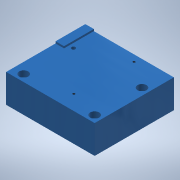
# Autodesk Inventor part: baseblock for AOTF
Saved by Autodesk Inventor 2022 (Build 260153000, 153)
## iProperties
Created: 2013-10-25
Part Number: baseblock for AOTF
Document SubType Name: Modeling
Designer: betzige
Density: 1 g/cm^3
Material: Generic
Appearance: Cyan
Author: betzige
Autodesk Inventor part; units mm, degrees
ref_plane "YZ Plane" through (0, 0, 0) normal (1, 0, 0) x (0, 1, 0)
ref_plane "XZ Plane" through (0, 0, 0) normal (0, 1, 0) x (-1, 0, 0)
ref_plane "XY Plane" through (0, 0, 0) normal (0, 0, 1) x (1, 0, 0)
sketch "Sketch1" plane through (0, 0, 0) normal (0, 0, 1) x (1, 0, 0)
  line L0 (-47.5, 42.5) -> (47.5, 42.5)
  line L1 (47.5, 42.5) -> (47.5, -42.5)
  line L2 (47.5, -42.5) -> (-47.5, -42.5)
  line L3 (-47.5, -42.5) -> (-47.5, 42.5)
  point P0 (0, 0)
  dimension "d0" = 95
  dimension "d1" = 85
  dimension "d2" = 47.5
  dimension "d3" = 42.5
  constraints: 8 end point, 2 parallel, 1 horizontal, 1 perpendicular
  measures "d0" distance of L0.start L0.end
  measures "d1" distance of L2.end L0.start
  measures "d2" distance from line of point (0, 0) L3
  measures "d3" distance from line of point (0, 0) L0
extrude "Extrusion1" add sketch "Sketch1" along normal blind 30.5168
sketch "Sketch2" plane through (0, 0, 30.5168) normal (0, 0, 1) x (1, 0, 0)
  arc A0 (-201.3, -568.6) -> (-188.8, -581.1) centre (-188.8, -568.6) ccw projected
  line L0 (-188.8, -581.1) -> (243.4, -581.1) projected
  arc A1 (243.4, -581.1) -> (255.9, -568.6) centre (243.4, -568.6) ccw projected
  line L1 (255.9, -568.6) -> (255.9, 16) projected
  arc A2 (255.9, 16) -> (243.4, 28.5) centre (243.4, 16) ccw projected
  line L2 (243.4, 28.5) -> (-188.8, 28.5) projected
  arc A3 (-188.8, 28.5) -> (-201.3, 16) centre (-188.8, 16) ccw projected
  line L3 (-201.3, 16) -> (-201.3, -568.6) projected
  circle A4 centre (217.8, -568.4) radius 2.5527 projected
  circle A5 centre (192.4, -568.4) radius 2.5527 projected
  circle A6 centre (167, -568.4) radius 2.5527 projected
  circle A7 centre (141.6, -568.4) radius 2.5527 projected
  circle A8 centre (116.2, -568.4) radius 2.5527 projected
  circle A9 centre (90.8, -568.4) radius 2.5527 projected
  circle A10 centre (65.4, -568.4) radius 2.5527 projected
  circle A11 centre (40, -568.4) radius 2.5527 projected
  circle A12 centre (14.6, -568.4) radius 2.5527 projected
  circle A13 centre (-10.8, -568.4) radius 2.5527 projected
  circle A14 centre (-36.2, -568.4) radius 2.5527 projected
  circle A15 centre (-61.6, -568.4) radius 2.5527 projected
  circle A16 centre (-87, -568.4) radius 2.5527 projected
  circle A17 centre (-112.4, -568.4) radius 2.5527 projected
  circle A18 centre (-137.8, -568.4) radius 2.5527 projected
  circle A19 centre (-163.2, -568.4) radius 2.5527 projected
  circle A20 centre (-188.6, -568.4) radius 2.5527 projected
  circle A21 centre (243.2, -543) radius 2.5527 projected
  circle A22 centre (217.8, -543) radius 2.5527 projected
  circle A23 centre (192.4, -543) radius 2.5527 projected
  circle A24 centre (167, -543) radius 2.5527 projected
  circle A25 centre (141.6, -543) radius 2.5527 projected
  circle A26 centre (116.2, -543) radius 2.5527 projected
  circle A27 centre (90.8, -543) radius 2.5527 projected
  circle A28 centre (65.4, -543) radius 2.5527 projected
  circle A29 centre (40, -543) radius 2.5527 projected
  circle A30 centre (14.6, -543) radius 2.5527 projected
  circle A31 centre (-10.8, -543) radius 2.5527 projected
  circle A32 centre (-36.2, -543) radius 2.5527 projected
  circle A33 centre (-61.6, -543) radius 2.5527 projected
  circle A34 centre (-87, -543) radius 2.5527 projected
  circle A35 centre (-112.4, -543) radius 2.5527 projected
  circle A36 centre (-137.8, -543) radius 2.5527 projected
  circle A37 centre (-163.2, -543) radius 2.5527 projected
  circle A38 centre (-188.6, -543) radius 2.5527 projected
  circle A39 centre (243.2, -517.6) radius 2.5527 projected
  circle A40 centre (217.8, -517.6) radius 2.5527 projected
  circle A41 centre (192.4, -517.6) radius 2.5527 projected
  circle A42 centre (167, -517.6) radius 2.5527 projected
  circle A43 centre (141.6, -517.6) radius 2.5527 projected
  circle A44 centre (116.2, -517.6) radius 2.5527 projected
  circle A45 centre (90.8, -517.6) radius 2.5527 projected
  circle A46 centre (65.4, -517.6) radius 2.5527 projected
  circle A47 centre (40, -517.6) radius 2.5527 projected
  circle A48 centre (14.6, -517.6) radius 2.5527 projected
  circle A49 centre (-10.8, -517.6) radius 2.5527 projected
  circle A50 centre (-36.2, -517.6) radius 2.5527 projected
  circle A51 centre (-61.6, -517.6) radius 2.5527 projected
  circle A52 centre (-87, -517.6) radius 2.5527 projected
  circle A53 centre (-112.4, -517.6) radius 2.5527 projected
  circle A54 centre (-137.8, -517.6) radius 2.5527 projected
  circle A55 centre (-163.2, -517.6) radius 2.5527 projected
  circle A56 centre (-188.6, -517.6) radius 2.5527 projected
  circle A57 centre (243.2, -492.2) radius 2.5527 projected
  circle A58 centre (217.8, -492.2) radius 2.5527 projected
  circle A59 centre (192.4, -492.2) radius 2.5527 projected
  circle A60 centre (167, -492.2) radius 2.5527 projected
  circle A61 centre (141.6, -492.2) radius 2.5527 projected
  circle A62 centre (116.2, -492.2) radius 2.5527 projected
  circle A63 centre (90.8, -492.2) radius 2.5527 projected
  circle A64 centre (65.4, -492.2) radius 2.5527 projected
  circle A65 centre (40, -492.2) radius 2.5527 projected
  circle A66 centre (14.6, -492.2) radius 2.5527 projected
  circle A67 centre (-10.8, -492.2) radius 2.5527 projected
  circle A68 centre (-36.2, -492.2) radius 2.5527 projected
  circle A69 centre (-61.6, -492.2) radius 2.5527 projected
  circle A70 centre (-87, -492.2) radius 2.5527 projected
  circle A71 centre (-112.4, -492.2) radius 2.5527 projected
  circle A72 centre (-137.8, -492.2) radius 2.5527 projected
  circle A73 centre (-163.2, -492.2) radius 2.5527 projected
  circle A74 centre (-188.6, -492.2) radius 2.5527 projected
  circle A75 centre (243.2, -466.8) radius 2.5527 projected
  circle A76 centre (217.8, -466.8) radius 2.5527 projected
  circle A77 centre (192.4, -466.8) radius 2.5527 projected
  circle A78 centre (167, -466.8) radius 2.5527 projected
  circle A79 centre (141.6, -466.8) radius 2.5527 projected
  circle A80 centre (116.2, -466.8) radius 2.5527 projected
  circle A81 centre (90.8, -466.8) radius 2.5527 projected
  circle A82 centre (65.4, -466.8) radius 2.5527 projected
  circle A83 centre (40, -466.8) radius 2.5527 projected
  circle A84 centre (14.6, -466.8) radius 2.5527 projected
  circle A85 centre (-10.8, -466.8) radius 2.5527 projected
  circle A86 centre (-36.2, -466.8) radius 2.5527 projected
  circle A87 centre (-61.6, -466.8) radius 2.5527 projected
  circle A88 centre (-87, -466.8) radius 2.5527 projected
  circle A89 centre (-112.4, -466.8) radius 2.5527 projected
  circle A90 centre (-137.8, -466.8) radius 2.5527 projected
  circle A91 centre (-163.2, -466.8) radius 2.5527 projected
  circle A92 centre (-188.6, -466.8) radius 2.5527 projected
  circle A93 centre (243.2, -441.4) radius 2.5527 projected
  circle A94 centre (217.8, -441.4) radius 2.5527 projected
  circle A95 centre (192.4, -441.4) radius 2.5527 projected
  circle A96 centre (167, -441.4) radius 2.5527 projected
  circle A97 centre (141.6, -441.4) radius 2.5527 projected
  circle A98 centre (116.2, -441.4) radius 2.5527 projected
  circle A99 centre (90.8, -441.4) radius 2.5527 projected
  circle A100 centre (65.4, -441.4) radius 2.5527 projected
  circle A101 centre (40, -441.4) radius 2.5527 projected
  circle A102 centre (14.6, -441.4) radius 2.5527 projected
  circle A103 centre (-10.8, -441.4) radius 2.5527 projected
  circle A104 centre (-36.2, -441.4) radius 2.5527 projected
  circle A105 centre (-61.6, -441.4) radius 2.5527 projected
  circle A106 centre (-87, -441.4) radius 2.5527 projected
  circle A107 centre (-112.4, -441.4) radius 2.5527 projected
  circle A108 centre (-137.8, -441.4) radius 2.5527 projected
  circle A109 centre (-163.2, -441.4) radius 2.5527 projected
  circle A110 centre (-188.6, -441.4) radius 2.5527 projected
  circle A111 centre (243.2, -416) radius 2.5527 projected
  circle A112 centre (217.8, -416) radius 2.5527 projected
  circle A113 centre (192.4, -416) radius 2.5527 projected
  circle A114 centre (167, -416) radius 2.5527 projected
  circle A115 centre (141.6, -416) radius 2.5527 projected
  circle A116 centre (116.2, -416) radius 2.5527 projected
  circle A117 centre (90.8, -416) radius 2.5527 projected
  circle A118 centre (65.4, -416) radius 2.5527 projected
  circle A119 centre (40, -416) radius 2.5527 projected
  circle A120 centre (14.6, -416) radius 2.5527 projected
  circle A121 centre (-10.8, -416) radius 2.5527 projected
  circle A122 centre (-36.2, -416) radius 2.5527 projected
  circle A123 centre (-61.6, -416) radius 2.5527 projected
  circle A124 centre (-87, -416) radius 2.5527 projected
  circle A125 centre (-112.4, -416) radius 2.5527 projected
  circle A126 centre (-137.8, -416) radius 2.5527 projected
  circle A127 centre (-163.2, -416) radius 2.5527 projected
  circle A128 centre (-188.6, -416) radius 2.5527 projected
  circle A129 centre (243.2, -390.6) radius 2.5527 projected
  circle A130 centre (217.8, -390.6) radius 2.5527 projected
  circle A131 centre (192.4, -390.6) radius 2.5527 projected
  circle A132 centre (167, -390.6) radius 2.5527 projected
  circle A133 centre (141.6, -390.6) radius 2.5527 projected
  circle A134 centre (116.2, -390.6) radius 2.5527 projected
  circle A135 centre (90.8, -390.6) radius 2.5527 projected
  circle A136 centre (65.4, -390.6) radius 2.5527 projected
  circle A137 centre (40, -390.6) radius 2.5527 projected
  circle A138 centre (14.6, -390.6) radius 2.5527 projected
  circle A139 centre (-10.8, -390.6) radius 2.5527 projected
  circle A140 centre (-36.2, -390.6) radius 2.5527 projected
  circle A141 centre (-61.6, -390.6) radius 2.5527 projected
  circle A142 centre (-87, -390.6) radius 2.5527 projected
  circle A143 centre (-112.4, -390.6) radius 2.5527 projected
  circle A144 centre (-137.8, -390.6) radius 2.5527 projected
  circle A145 centre (-163.2, -390.6) radius 2.5527 projected
  circle A146 centre (-188.6, -390.6) radius 2.5527 projected
  circle A147 centre (243.2, -365.2) radius 2.5527 projected
  circle A148 centre (217.8, -365.2) radius 2.5527 projected
  circle A149 centre (192.4, -365.2) radius 2.5527 projected
  circle A150 centre (167, -365.2) radius 2.5527 projected
  circle A151 centre (141.6, -365.2) radius 2.5527 projected
  circle A152 centre (116.2, -365.2) radius 2.5527 projected
  circle A153 centre (90.8, -365.2) radius 2.5527 projected
  circle A154 centre (65.4, -365.2) radius 2.5527 projected
  circle A155 centre (40, -365.2) radius 2.5527 projected
  circle A156 centre (14.6, -365.2) radius 2.5527 projected
  circle A157 centre (-10.8, -365.2) radius 2.5527 projected
  circle A158 centre (-36.2, -365.2) radius 2.5527 projected
  circle A159 centre (-61.6, -365.2) radius 2.5527 projected
  circle A160 centre (-87, -365.2) radius 2.5527 projected
  circle A161 centre (-112.4, -365.2) radius 2.5527 projected
  circle A162 centre (-137.8, -365.2) radius 2.5527 projected
  circle A163 centre (-163.2, -365.2) radius 2.5527 projected
  circle A164 centre (-188.6, -365.2) radius 2.5527 projected
  circle A165 centre (243.2, -339.8) radius 2.5527 projected
  circle A166 centre (217.8, -339.8) radius 2.5527 projected
  circle A167 centre (192.4, -339.8) radius 2.5527 projected
  circle A168 centre (167, -339.8) radius 2.5527 projected
  circle A169 centre (141.6, -339.8) radius 2.5527 projected
  circle A170 centre (116.2, -339.8) radius 2.5527 projected
  circle A171 centre (90.8, -339.8) radius 2.5527 projected
  circle A172 centre (65.4, -339.8) radius 2.5527 projected
  circle A173 centre (40, -339.8) radius 2.5527 projected
  circle A174 centre (14.6, -339.8) radius 2.5527 projected
  circle A175 centre (-10.8, -339.8) radius 2.5527 projected
  circle A176 centre (-36.2, -339.8) radius 2.5527 projected
  circle A177 centre (-61.6, -339.8) radius 2.5527 projected
  circle A178 centre (-87, -339.8) radius 2.5527 projected
  circle A179 centre (-112.4, -339.8) radius 2.5527 projected
  circle A180 centre (-137.8, -339.8) radius 2.5527 projected
  circle A181 centre (-163.2, -339.8) radius 2.5527 projected
  circle A182 centre (-188.6, -339.8) radius 2.5527 projected
  circle A183 centre (243.2, -314.4) radius 2.5527 projected
  circle A184 centre (217.8, -314.4) radius 2.5527 projected
  circle A185 centre (192.4, -314.4) radius 2.5527 projected
  circle A186 centre (167, -314.4) radius 2.5527 projected
  circle A187 centre (141.6, -314.4) radius 2.5527 projected
  circle A188 centre (116.2, -314.4) radius 2.5527 projected
  circle A189 centre (90.8, -314.4) radius 2.5527 projected
  circle A190 centre (65.4, -314.4) radius 2.5527 projected
  circle A191 centre (40, -314.4) radius 2.5527 projected
  circle A192 centre (14.6, -314.4) radius 2.5527 projected
  circle A193 centre (-10.8, -314.4) radius 2.5527 projected
  circle A194 centre (-36.2, -314.4) radius 2.5527 projected
  circle A195 centre (-61.6, -314.4) radius 2.5527 projected
  circle A196 centre (-87, -314.4) radius 2.5527 projected
  circle A197 centre (-112.4, -314.4) radius 2.5527 projected
  circle A198 centre (-137.8, -314.4) radius 2.5527 projected
  circle A199 centre (-163.2, -314.4) radius 2.5527 projected
  circle A200 centre (-188.6, -314.4) radius 2.5527 projected
  circle A201 centre (243.2, -289) radius 2.5527 projected
  circle A202 centre (217.8, -289) radius 2.5527 projected
  circle A203 centre (192.4, -289) radius 2.5527 projected
  circle A204 centre (167, -289) radius 2.5527 projected
  circle A205 centre (141.6, -289) radius 2.5527 projected
  circle A206 centre (116.2, -289) radius 2.5527 projected
  circle A207 centre (90.8, -289) radius 2.5527 projected
  circle A208 centre (65.4, -289) radius 2.5527 projected
  circle A209 centre (40, -289) radius 2.5527 projected
  circle A210 centre (14.6, -289) radius 2.5527 projected
  circle A211 centre (-10.8, -289) radius 2.5527 projected
  circle A212 centre (-36.2, -289) radius 2.5527 projected
  circle A213 centre (-61.6, -289) radius 2.5527 projected
  circle A214 centre (-87, -289) radius 2.5527 projected
  circle A215 centre (-112.4, -289) radius 2.5527 projected
  circle A216 centre (-137.8, -289) radius 2.5527 projected
  circle A217 centre (-163.2, -289) radius 2.5527 projected
  circle A218 centre (-188.6, -289) radius 2.5527 projected
  circle A219 centre (243.2, -263.6) radius 2.5527 projected
  circle A220 centre (217.8, -263.6) radius 2.5527 projected
  circle A221 centre (192.4, -263.6) radius 2.5527 projected
  circle A222 centre (167, -263.6) radius 2.5527 projected
  circle A223 centre (141.6, -263.6) radius 2.5527 projected
  circle A224 centre (116.2, -263.6) radius 2.5527 projected
  circle A225 centre (90.8, -263.6) radius 2.5527 projected
  circle A226 centre (65.4, -263.6) radius 2.5527 projected
  circle A227 centre (40, -263.6) radius 2.5527 projected
  circle A228 centre (14.6, -263.6) radius 2.5527 projected
  circle A229 centre (-10.8, -263.6) radius 2.5527 projected
  circle A230 centre (-36.2, -263.6) radius 2.5527 projected
  circle A231 centre (-61.6, -263.6) radius 2.5527 projected
  circle A232 centre (-87, -263.6) radius 2.5527 projected
  circle A233 centre (-112.4, -263.6) radius 2.5527 projected
  circle A234 centre (-137.8, -263.6) radius 2.5527 projected
  circle A235 centre (-163.2, -263.6) radius 2.5527 projected
  circle A236 centre (-188.6, -263.6) radius 2.5527 projected
  circle A237 centre (243.2, -238.2) radius 2.5527 projected
  circle A238 centre (217.8, -238.2) radius 2.5527 projected
  circle A239 centre (192.4, -238.2) radius 2.5527 projected
  circle A240 centre (167, -238.2) radius 2.5527 projected
  circle A241 centre (141.6, -238.2) radius 2.5527 projected
  circle A242 centre (116.2, -238.2) radius 2.5527 projected
  circle A243 centre (90.8, -238.2) radius 2.5527 projected
  circle A244 centre (65.4, -238.2) radius 2.5527 projected
  circle A245 centre (40, -238.2) radius 2.5527 projected
  circle A246 centre (14.6, -238.2) radius 2.5527 projected
  circle A247 centre (-10.8, -238.2) radius 2.5527 projected
  circle A248 centre (-36.2, -238.2) radius 2.5527 projected
  circle A249 centre (-61.6, -238.2) radius 2.5527 projected
  circle A250 centre (-87, -238.2) radius 2.5527 projected
  circle A251 centre (-112.4, -238.2) radius 2.5527 projected
  circle A252 centre (-137.8, -238.2) radius 2.5527 projected
  circle A253 centre (-163.2, -238.2) radius 2.5527 projected
  circle A254 centre (-188.6, -238.2) radius 2.5527 projected
  circle A255 centre (243.2, -212.8) radius 2.5527 projected
  circle A256 centre (217.8, -212.8) radius 2.5527 projected
  circle A257 centre (192.4, -212.8) radius 2.5527 projected
  circle A258 centre (167, -212.8) radius 2.5527 projected
  circle A259 centre (141.6, -212.8) radius 2.5527 projected
  circle A260 centre (116.2, -212.8) radius 2.5527 projected
  circle A261 centre (90.8, -212.8) radius 2.5527 projected
  circle A262 centre (65.4, -212.8) radius 2.5527 projected
  circle A263 centre (40, -212.8) radius 2.5527 projected
  circle A264 centre (14.6, -212.8) radius 2.5527 projected
  circle A265 centre (-10.8, -212.8) radius 2.5527 projected
  circle A266 centre (-36.2, -212.8) radius 2.5527 projected
  circle A267 centre (-61.6, -212.8) radius 2.5527 projected
  circle A268 centre (-87, -212.8) radius 2.5527 projected
  circle A269 centre (-112.4, -212.8) radius 2.5527 projected
  circle A270 centre (-137.8, -212.8) radius 2.5527 projected
  circle A271 centre (-163.2, -212.8) radius 2.5527 projected
  circle A272 centre (-188.6, -212.8) radius 2.5527 projected
  circle A273 centre (243.2, -187.4) radius 2.5527 projected
  circle A274 centre (217.8, -187.4) radius 2.5527 projected
  circle A275 centre (192.4, -187.4) radius 2.5527 projected
  circle A276 centre (167, -187.4) radius 2.5527 projected
  circle A277 centre (141.6, -187.4) radius 2.5527 projected
  circle A278 centre (116.2, -187.4) radius 2.5527 projected
  circle A279 centre (90.8, -187.4) radius 2.5527 projected
  circle A280 centre (65.4, -187.4) radius 2.5527 projected
  circle A281 centre (40, -187.4) radius 2.5527 projected
  circle A282 centre (14.6, -187.4) radius 2.5527 projected
  circle A283 centre (-10.8, -187.4) radius 2.5527 projected
  circle A284 centre (-36.2, -187.4) radius 2.5527 projected
  circle A285 centre (-61.6, -187.4) radius 2.5527 projected
  circle A286 centre (-87, -187.4) radius 2.5527 projected
  circle A287 centre (-112.4, -187.4) radius 2.5527 projected
  circle A288 centre (-137.8, -187.4) radius 2.5527 projected
  circle A289 centre (-163.2, -187.4) radius 2.5527 projected
  circle A290 centre (-188.6, -187.4) radius 2.5527 projected
  circle A291 centre (243.2, -162) radius 2.5527 projected
  circle A292 centre (217.8, -162) radius 2.5527 projected
  circle A293 centre (192.4, -162) radius 2.5527 projected
  circle A294 centre (167, -162) radius 2.5527 projected
  circle A295 centre (141.6, -162) radius 2.5527 projected
  circle A296 centre (116.2, -162) radius 2.5527 projected
  circle A297 centre (90.8, -162) radius 2.5527 projected
  circle A298 centre (65.4, -162) radius 2.5527 projected
  circle A299 centre (40, -162) radius 2.5527 projected
  circle A300 centre (14.6, -162) radius 2.5527 projected
  circle A301 centre (-10.8, -162) radius 2.5527 projected
  circle A302 centre (-36.2, -162) radius 2.5527 projected
  circle A303 centre (-61.6, -162) radius 2.5527 projected
  circle A304 centre (-87, -162) radius 2.5527 projected
  circle A305 centre (-112.4, -162) radius 2.5527 projected
  circle A306 centre (-137.8, -162) radius 2.5527 projected
  circle A307 centre (-163.2, -162) radius 2.5527 projected
  circle A308 centre (-188.6, -162) radius 2.5527 projected
  circle A309 centre (243.2, -136.6) radius 2.5527 projected
  circle A310 centre (217.8, -136.6) radius 2.5527 projected
  circle A311 centre (192.4, -136.6) radius 2.5527 projected
  circle A312 centre (167, -136.6) radius 2.5527 projected
  circle A313 centre (141.6, -136.6) radius 2.5527 projected
  circle A314 centre (116.2, -136.6) radius 2.5527 projected
  circle A315 centre (90.8, -136.6) radius 2.5527 projected
  circle A316 centre (65.4, -136.6) radius 2.5527 projected
  circle A317 centre (40, -136.6) radius 2.5527 projected
  circle A318 centre (14.6, -136.6) radius 2.5527 projected
  circle A319 centre (-10.8, -136.6) radius 2.5527 projected
  circle A320 centre (-36.2, -136.6) radius 2.5527 projected
  circle A321 centre (-61.6, -136.6) radius 2.5527 projected
  circle A322 centre (-87, -136.6) radius 2.5527 projected
  circle A323 centre (-112.4, -136.6) radius 2.5527 projected
  circle A324 centre (-137.8, -136.6) radius 2.5527 projected
  circle A325 centre (-163.2, -136.6) radius 2.5527 projected
  circle A326 centre (-188.6, -136.6) radius 2.5527 projected
  circle A327 centre (243.2, -111.2) radius 2.5527 projected
  circle A328 centre (217.8, -111.2) radius 2.5527 projected
  circle A329 centre (192.4, -111.2) radius 2.5527 projected
  circle A330 centre (167, -111.2) radius 2.5527 projected
  circle A331 centre (141.6, -111.2) radius 2.5527 projected
  circle A332 centre (116.2, -111.2) radius 2.5527 projected
  circle A333 centre (90.8, -111.2) radius 2.5527 projected
  circle A334 centre (65.4, -111.2) radius 2.5527 projected
  circle A335 centre (40, -111.2) radius 2.5527 projected
  circle A336 centre (14.6, -111.2) radius 2.5527 projected
  circle A337 centre (-10.8, -111.2) radius 2.5527 projected
  circle A338 centre (-36.2, -111.2) radius 2.5527 projected
  circle A339 centre (-61.6, -111.2) radius 2.5527 projected
  circle A340 centre (-87, -111.2) radius 2.5527 projected
  circle A341 centre (-112.4, -111.2) radius 2.5527 projected
  circle A342 centre (-137.8, -111.2) radius 2.5527 projected
  circle A343 centre (-163.2, -111.2) radius 2.5527 projected
  circle A344 centre (-188.6, -111.2) radius 2.5527 projected
  circle A345 centre (243.2, -85.8) radius 2.5527 projected
  circle A346 centre (217.8, -85.8) radius 2.5527 projected
  circle A347 centre (192.4, -85.8) radius 2.5527 projected
  circle A348 centre (167, -85.8) radius 2.5527 projected
  circle A349 centre (141.6, -85.8) radius 2.5527 projected
  circle A350 centre (116.2, -85.8) radius 2.5527 projected
  circle A351 centre (90.8, -85.8) radius 2.5527 projected
  circle A352 centre (65.4, -85.8) radius 2.5527 projected
  circle A353 centre (40, -85.8) radius 2.5527 projected
  circle A354 centre (14.6, -85.8) radius 2.5527 projected
  circle A355 centre (-10.8, -85.8) radius 2.5527 projected
  circle A356 centre (-36.2, -85.8) radius 2.5527 projected
  circle A357 centre (-61.6, -85.8) radius 2.5527 projected
  circle A358 centre (-87, -85.8) radius 2.5527 projected
  circle A359 centre (-112.4, -85.8) radius 2.5527 projected
  circle A360 centre (-137.8, -85.8) radius 2.5527 projected
  circle A361 centre (-163.2, -85.8) radius 2.5527 projected
  circle A362 centre (-188.6, -85.8) radius 2.5527 projected
  circle A363 centre (243.2, -60.4) radius 2.5527 projected
  circle A364 centre (217.8, -60.4) radius 2.5527 projected
  circle A365 centre (192.4, -60.4) radius 2.5527 projected
  circle A366 centre (167, -60.4) radius 2.5527 projected
  circle A367 centre (141.6, -60.4) radius 2.5527 projected
  circle A368 centre (116.2, -60.4) radius 2.5527 projected
  circle A369 centre (90.8, -60.4) radius 2.5527 projected
  circle A370 centre (65.4, -60.4) radius 2.5527 projected
  circle A371 centre (40, -60.4) radius 2.5527 projected
  circle A372 centre (14.6, -60.4) radius 2.5527 projected
  circle A373 centre (-10.8, -60.4) radius 2.5527 projected
  circle A374 centre (-36.2, -60.4) radius 2.5527 projected
  circle A375 centre (-61.6, -60.4) radius 2.5527 projected
  circle A376 centre (-87, -60.4) radius 2.5527 projected
  circle A377 centre (-112.4, -60.4) radius 2.5527 projected
  circle A378 centre (-137.8, -60.4) radius 2.5527 projected
  circle A379 centre (-163.2, -60.4) radius 2.5527 projected
  circle A380 centre (-188.6, -60.4) radius 2.5527 projected
  circle A381 centre (243.2, -35) radius 2.5527 projected
  circle A382 centre (217.8, -35) radius 2.5527 projected
  circle A383 centre (192.4, -35) radius 2.5527 projected
  circle A384 centre (167, -35) radius 2.5527 projected
  circle A385 centre (141.6, -35) radius 2.5527 projected
  circle A386 centre (116.2, -35) radius 2.5527 projected
  circle A387 centre (90.8, -35) radius 2.5527 projected
  circle A388 centre (65.4, -35) radius 2.5527 projected
  circle A389 centre (40, -35) radius 2.5527 projected
  circle A390 centre (14.6, -35) radius 2.5527 projected
  circle A391 centre (-10.8, -35) radius 2.5527 projected
  circle A392 centre (-36.2, -35) radius 2.5527 projected
  circle A393 centre (-61.6, -35) radius 2.5527 projected
  circle A394 centre (-87, -35) radius 2.5527 projected
  circle A395 centre (-112.4, -35) radius 2.5527 projected
  circle A396 centre (-137.8, -35) radius 2.5527 projected
  circle A397 centre (-163.2, -35) radius 2.5527 projected
  circle A398 centre (-188.6, -35) radius 2.5527 projected
  circle A399 centre (243.2, -9.6) radius 2.5527 projected
  circle A400 centre (217.8, -9.6) radius 2.5527 projected
  circle A401 centre (192.4, -9.6) radius 2.5527 projected
  circle A402 centre (167, -9.6) radius 2.5527 projected
  circle A403 centre (141.6, -9.6) radius 2.5527 projected
  circle A404 centre (116.2, -9.6) radius 2.5527 projected
  circle A405 centre (90.8, -9.6) radius 2.5527 projected
  circle A406 centre (65.4, -9.6) radius 2.5527 projected
  circle A407 centre (40, -9.6) radius 2.5527 projected
  circle A408 centre (14.6, -9.6) radius 2.5527 projected
  circle A409 centre (-10.8, -9.6) radius 2.5527 projected
  circle A410 centre (-36.2, -9.6) radius 2.5527 projected
  circle A411 centre (-61.6, -9.6) radius 2.5527 projected
  circle A412 centre (-87, -9.6) radius 2.5527 projected
  circle A413 centre (-112.4, -9.6) radius 2.5527 projected
  circle A414 centre (-137.8, -9.6) radius 2.5527 projected
  circle A415 centre (-163.2, -9.6) radius 2.5527 projected
  circle A416 centre (-188.6, -9.6) radius 2.5527 projected
  circle A417 centre (243.2, 15.8) radius 2.5527 projected
  circle A418 centre (217.8, 15.8) radius 2.5527 projected
  circle A419 centre (192.4, 15.8) radius 2.5527 projected
  circle A420 centre (167, 15.8) radius 2.5527 projected
  circle A421 centre (141.6, 15.8) radius 2.5527 projected
  circle A422 centre (116.2, 15.8) radius 2.5527 projected
  circle A423 centre (90.8, 15.8) radius 2.5527 projected
  circle A424 centre (65.4, 15.8) radius 2.5527 projected
  circle A425 centre (40, 15.8) radius 2.5527 projected
  circle A426 centre (14.6, 15.8) radius 2.5527 projected
  circle A427 centre (-10.8, 15.8) radius 2.5527 projected
  circle A428 centre (-36.2, 15.8) radius 2.5527 projected
  circle A429 centre (-61.6, 15.8) radius 2.5527 projected
  circle A430 centre (-87, 15.8) radius 2.5527 projected
  circle A431 centre (-112.4, 15.8) radius 2.5527 projected
  circle A432 centre (-137.8, 15.8) radius 2.5527 projected
  circle A433 centre (-163.2, 15.8) radius 2.5527 projected
  circle A434 centre (-188.6, 15.8) radius 2.5527 projected
  circle A435 centre (243.2, -568.4) radius 2.5527 projected
  point P0 (0, 0)
  constraints: 3 coincident
hole "Hole1" at (40, 15.8, 30.5168) at (40, -35, 30.5168) at (-36.2, -35, 30.5168) direction (0, 0, -1) diameter 6.35 end through all counterbore diameter 9.652 counterbore depth 6.5
sketch "Sketch3" plane through (0, 0, 30.5168) normal (0, 0, 1) x (1, 0, 0)
  line L0 (26.7983, -23.1663) -> (-8.171, -21.7006) projected
  line L1 (-8.506, -29.6936) -> (-8.171, -21.7006) projected
  line L2 (26.4633, -31.1592) -> (-8.506, -29.6936) projected
  line L3 (26.7983, -23.1663) -> (26.4633, -31.1592) projected
  circle A0 centre (9.1461, -26.4299) radius 1.75 projected
  line L4 (-5.9098, 32.252) -> (29.0595, 30.7864) projected
  line L5 (29.3946, 38.7794) -> (29.0595, 30.7864) projected
  line L6 (-5.5747, 40.245) -> (29.3946, 38.7794) projected
  line L7 (-5.9098, 32.252) -> (-5.5747, 40.245) projected
  circle A1 centre (11.7424, 35.5157) radius 1.75 projected
  point P0 (0, 0)
  constraints: 2 coincident
hole "Hole2" at (9.1461, -26.4299, 30.5168) at (11.7424, 35.5157, 30.5168) direction (0, 0, -1) diameter 2.459 depth 6 tip angle 118 thread size "M3x0.5" class "6H" standard "ANSI Metric M Profile"
sketch "Sketch4" plane through (0, 0, 0) normal (0, 0, -1) x (-1, 0, 0)
  circle A0 centre (33.5506, 15.8) radius 2.3368 projected
  point P0 (0, 0)
hole "Hole3" at (-33.5506, 15.8, 0) direction (0, 0, 1) diameter 4.1656 end through all counterbore diameter 7.112 counterbore depth 24
sketch "Sketch5" plane through (0, 0, 30.5168) normal (0, 0, 1) x (1, 0, 0)
  line L0 (-47.5, 42.5) -> (47.5, 42.5) projected
  line L1 (-47.5, -42.5) -> (-47.5, 42.5) projected
  line L2 (-38.3766, 10.7023) -> (-38.3766, 20.8977) projected
  line L3 (-38.3766, 42.5) -> (-47.5, 42.5)
  line L4 (-47.5, 42.5) -> (-47.5, 10.5)
  line L5 (-47.5, 10.5) -> (-38.3766, 10.5)
  line L6 (-38.3766, 10.5) -> (-38.3766, 42.5)
  point P0 (0, 0)
  dimension "d27" = 32
  constraints: 8 end point, 2 parallel, 2 point on line, 1 horizontal, 1 perpendicular
  measures "d27" distance between parallel lines of L0 L5
extrude "Extrusion2" add sketch "Sketch5" along normal blind 2
body "Solid1"
